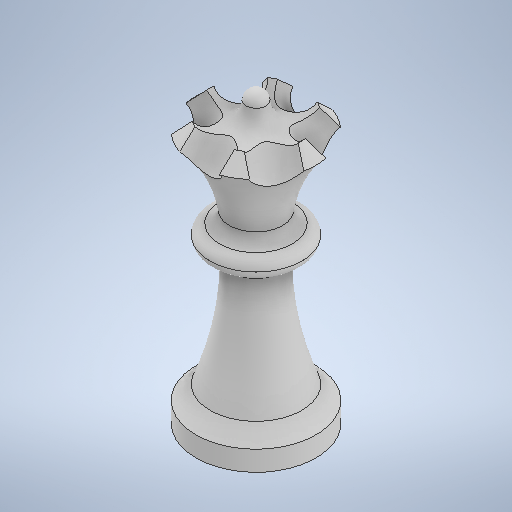
# Autodesk Inventor part: PawnUntagged
Saved by Autodesk Inventor 2025.2 (Build 292293000, 293)
## iProperties
Created: 2025-02-26
Part Number: PawnUntagged
Material: Generic
Document SubType Name: Modeling
Designer: Marcu
Density: 1 g/cm^3
Appearance: Default
Author: Marcu
Autodesk Inventor part; units mm, degrees
ref_plane "YZ Plane" through (0, 0, 0) normal (1, 0, 0) x (0, 1, 0)
ref_plane "XZ Plane" through (0, 0, 0) normal (0, 1, 0) x (-1, 0, 0)
ref_plane "XY Plane" through (0, 0, 0) normal (0, 0, 1) x (1, 0, 0)
sketch "Sketch1" plane through (0, 0, 0) normal (1, 0, 0) x (0, 1, 0)
  line L0 (4, 0) -> (4, 2.5)
  line L1 (4, 2.5) -> (0, 2.5)
  line L2 (0, 2.5) -> (0, 15)
  line L3 (0, 15) -> (5, 15)
  line L4 (5, 15) -> (8.5355, 11.4645)
  line L5 (38.3857, 6.4645) -> (38.3857, 11.4667)
  line L6 (38.3857, 11.4667) -> (43.3857, 11.4667)
  line L7 (43.3857, 11.4667) -> (43.3857, 6.4667)
  line L8 (63.3857, 15.0022) -> (66.9213, 11.4667)
  arc A0 (43.3857, 6.4667) -> (63.3857, 15.0022) centre (42.4106, 36.4509) ccw
  line L9 (0, 0) -> (72.5, 0)
  arc A1 (66.9213, 11.4667) -> (70, 2.5) centre (70, 7.5119) ccw
  line L10 (70, 2.5) -> (72.5, 2.5)
  line L11 (72.5, 2.5) -> (72.5, 0)
  arc A2 (8.5355, 11.4645) -> (38.3857, 6.4645) centre (35.5959, 81.4126) ccw
  dimension "d48" = 2.5
  dimension "d0" = 4
  dimension "d1" = 2.5
  dimension "d2" = 15
  dimension "d3" = 5
  dimension "d4" = 5
  dimension "d5" = 135
  dimension "d36" = 5
  dimension "d37" = 5
  dimension "d39" = 20
  dimension "d40" = 30
  dimension "d45" = 2.5
  dimension "d46" = 75
  constraints: 24 end point, 6 point on circle, 4 perpendicular, 3 centre point, 3 horizontal, 2 vertical
  measures "d0" distance of L9.start L0.start
  measures "d1" distance of L0.start L0.end
  measures "d2" distance of L9.start L2.end
  measures "d3" distance of L2.end L3.end
  measures "d4" distance of L3.end L4.end
  measures "d5" angle of L3 L4
  measures "d36" distance of L5.end L6.end
  measures "d37" distance of L8.start L8.end
  measures "d39" horizontal distance of L7.end L8.start
  measures "d40" radius of A0
  measures "d45" distance of L10.start L10.end
  measures "d46" radius of A2
revolve "Revolution1" add sketch "Sketch1" angle 360 about axis through (0, 0, 0) along (0, 1, 0)
fillet "Fillet1" radius 2.5 5 edges at (0, 43.3857, -6.4667) (0, 43.3857, -11.4667) (0, 38.3857, -11.4667) (0, 38.3857, -6.4645) (0, 72.5, -2.5)
sketch "Sketch2" plane through (0, 0, 0) normal (1, 0, 0) x (0, 1, 0)
  line L0 (66.9213, -11.4667) -> (66.9213, 11.4667) projected
  line L1 (63.3857, -15.0022) -> (63.3857, 15.0022) projected
  line L2 (69.0426, 9.3454) -> (72.5781, 12.8809)
  line L3 (72.5781, 12.8809) -> (64.7999, 20.6591)
  line L4 (64.7999, 20.6591) -> (61.2644, 17.1236)
  line L5 (69.0426, 9.3454) -> (61.2644, 17.1236)
  point P0 (0, 0)
  dimension "d50" = 8
  dimension "d51" = 5
  dimension "d52" = 11
  constraints: 8 end point, 1 perpendicular
  measures "d50" distance of L1.end L2.start
  measures "d51" distance of L2.start L2.end
  measures "d52" distance of L2.end L3.end
revolve "Revolution2" cut sketch "Sketch2" angle 360 about axis through (0, 69.0426, 9.3454) along (0, -0.7071068, 0.7071068)
pattern_circular "Circular Pattern1" count 6 over 360 about axis through (0, -10, 0) along (0, 1, 0) of "Revolution2"
body "Solid1"
